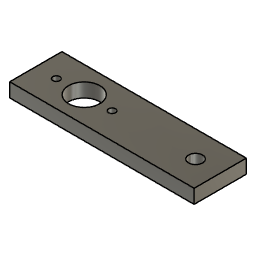
Verbindung Lenkmotor v3 (Autodesk Fusion 360 design; units mm, degrees)
Autodesk Fusion 360 part; units mm, degrees
note: some values were not read from the file. Chosen so that the rebuilt part matches the saved one: which face or edge a step refers to. Set by a fixed rule: which sketch regions a step uses.
sketch "Skizze1" plane through (0, 0, 0) normal (0, 0, 1) x (1, 0, 0)
  line L0 (0, 0) -> (80, 0)
  line L1 (80, 0) -> (80, 15)
  line L2 (80, 15) -> (0, 15)
  line L3 (0, 15) -> (0, 0)
  circle A0 centre (5.9189, 7.5) radius 1
  circle A1 centre (13.9189, 7.5) radius 4.5
  circle A2 centre (45.9189, 7.5) radius 2
  circle A3 centre (21.9189, 7.5) radius 1
  dimension "d1" = 80
  dimension "d2" = 2
  dimension "d4" = 9
  dimension "d6" = 4
  dimension "d7" = 2
  constraint horizontal L0
  constraint vertical L1
  constraint horizontal L2
  constraint vertical L3
  constraint coincident L0.start L3.end
  measures "d1" distance of L0.start L0.end
  measures "d2" diameter of A0
  measures "d4" diameter of A1
  measures "d6" diameter of A2
  measures "d7" diameter of A3
extrude "Extrusion1" add sketch "Skizze1" along normal blind 2
sketch "Skizze2" plane through (0, 0, 2) normal (0, 0, 1) x (-1, 0, 0)
  circle A0 centre (-13.9189, -7.5) radius 4.5
  circle A1 centre (-21.9189, -7.5) radius 1
  circle A2 centre (-5.9189, -7.5) radius 1
  circle A3 centre (-45.9189, -7.5) radius 2
  line L0 (0, -15) -> (0, 0)
  line L1 (0, 0) -> (-80, 0)
  line L2 (-80, 0) -> (-80, -15)
  line L3 (-80, -15) -> (0, -15)
sketch "Skizze3" plane through (0, 0, 2) normal (0, 0, 1) x (-1, 0, 0)
  circle A0 centre (-32.5, -7.5) radius 2
  line L0 (-32.4606, -9.4996) -> (-73.9606, -9.4996)
  line L1 (-73.9606, -9.4996) -> (-73.9606, -5.4996)
  line L2 (-73.9606, -5.4996) -> (-32.4606, -5.4996)
  line L3 (-32.4606, -5.4996) -> (-32.4606, -9.4996)
  dimension "d11" = 4
  dimension "d12" = 41.5
  dimension "d13" = 41.5
  dimension "d14" = 41.5
  dimension "d15" = 90
  dimension "d16" = 4
  constraint horizontal L0
  constraint vertical L1
  constraint horizontal L2
  constraint vertical L3
  constraint coincident A0 L0.start
  measures "d11" diameter of A0
  measures "d12" distance of L1.end L2.end
  measures "d13" distance of L1.end L2.end
  measures "d14" distance of L1.end L2.end
  measures "d15" angle of L0 L3
  measures "d16" distance of L0.start L2.end
extrude "Extrusion2" cut sketch "Skizze3" against normal blind 2
delete_face "Fläche löschen1" 6 faces at (45.9495, 9.4998, 1.3333) (36.9336, 9.4996, 1.3333) (32.3623, 5.5047, 0.6667) (60.1273, 5.4996, 1.3333) (73.9606, 8.1663, 1.3333) (55.2924, 9.4996, 1.3333)
sketch "Skizze4" plane through (0, 0, 2) normal (0, 0, 1) x (-1, 0, 0)
extrude "Extrusion3" cut sketch "Skizze2" against normal blind 2 contours A3
extrude "Extrusion4" add 1 faces at (69.3063, 7.5, 2) along direction (0, 0, 1) blind 2
sketch "Skizze5" plane through (0, 0, 4) normal (0, 0, 1) x (-1, 0, 0)
  circle A0 centre (-45.9189, -7.5) radius 2
  circle A1 centre (-5.9189, -7.5) radius 1
  circle A2 centre (-13.9189, -7.5) radius 4.5
  circle A3 centre (-21.9189, -7.5) radius 1
  line L0 (0, -15) -> (0, 0)
  line L1 (0, 0) -> (-80, 0)
  line L2 (-80, 0) -> (-80, -15)
  line L3 (-80, -15) -> (0, -15)
  line L4 (-53, -15) -> (-80, -15)
  line L5 (-80, -15) -> (-80, 0)
  line L6 (-80, 0) -> (-53, 0)
  line L7 (-53, 0) -> (-53, -15)
  constraint horizontal L4
  constraint vertical L5
  constraint horizontal L6
  constraint vertical L7
  constraint coincident L1.end L2.start
  constraint coincident L3 L4.start
extrude "Extrusion5" cut sketch "Skizze5" against normal blind 10 contours L1 L2 L3 L4 L5 L6 L7
